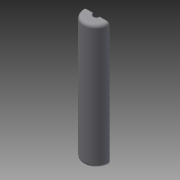
# Autodesk Inventor part: Wagon Hand Handle V03
Saved by Autodesk Inventor 2014 (Build 180170000, 170)
## iProperties
Created: 2013-11-30
Part Number: Wagon Hand Handle V03
Material: Generic
Document SubType Name: Modeling
Designer: steele
Density: 1 g/cm^3
Appearance: Default
Author: steele
Autodesk Inventor part; units mm, degrees
ref_plane "YZ Plane" through (0, 0, 0) normal (1, 0, 0) x (0, 1, 0)
ref_plane "XZ Plane" through (0, 0, 0) normal (0, 1, 0) x (-1, 0, 0)
ref_plane "XY Plane" through (0, 0, 0) normal (0, 0, 1) x (1, 0, 0)
sketch "Sketch1" plane through (0, 0, 0) normal (0, 0, 1) x (1, 0, 0)
  circle A0 centre (0, 0) radius 12.7
  circle A1 centre (0, 0) radius 3.302
  dimension "d0" = 25.4
  dimension "d1" = 6.604
  constraints: 2 centre point, 2 coincident
  measures "d0" diameter of A0
  measures "d1" diameter of A1
extrude "Extrusion1" add sketch "Sketch1" along normal mid plane 120.65
fillet "Fillet1" radius 3 2 edges at (-12.7, 0, 60.325) (-12.7, 0, -60.325)
sketch "Sketch3" plane through (0, 0, 60.325) normal (0, 0, 1) x (1, 0, 0)
  line L0 (-31, 0) -> (39, 0)
  line L1 (39, 0) -> (17, 30)
  line L2 (17, 30) -> (-16, 29)
  line L3 (-16, 29) -> (-31, 0)
  constraints: 8 end point, 1 horizontal
extrude "Extrusion2" cut sketch "Sketch3" against normal through all
body "Solid1"
